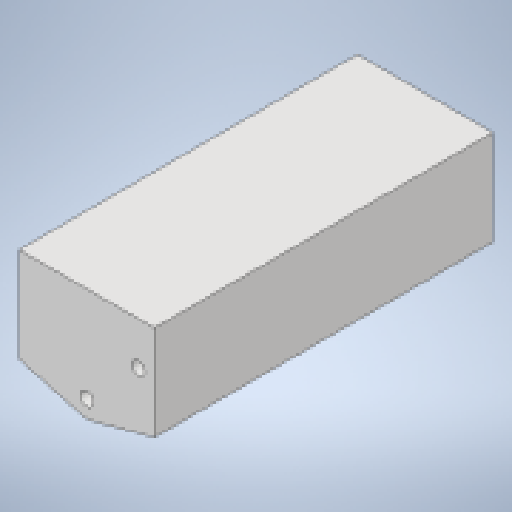
# Autodesk Inventor part: Корпус
Saved by Autodesk Inventor 2025 (Build 290162010, 162A)
## iProperties
Created: 2024-06-14
Part Number: Корпус
Material: Типовые
Document SubType Name: Modeling
Designer: Edward_Higgins
Density: 1 g/cm^3
Appearance: По умолчанию
Author: Edward_Higgins
Autodesk Inventor part; units mm, degrees
ref_plane "YZ Plane" through (0, 0, 0) normal (1, 0, 0) x (0, 1, 0)
ref_plane "XZ Plane" through (0, 0, 0) normal (0, 1, 0) x (-1, 0, 0)
ref_plane "XY Plane" through (0, 0, 0) normal (0, 0, 1) x (1, 0, 0)
sketch "Эскиз1" plane through (0, 0, 0) normal (0, 0, 1) x (1, 0, 0)
  line L0 (-50, 70) -> (50, 70)
  line L1 (50, 70) -> (50, 0)
  line L2 (50, 0) -> (-50, 0) construction
  line L3 (-50, 0) -> (-50, 70)
  circle A0 centre (0, 0) radius 5
  circle A1 centre (38.1838, 38.1838) radius 5
  line L4 (0, 0) -> (38.1838, 38.1838) construction
  line L5 (-50, 0) -> (-3.3494, -12.5)
  arc A2 (-3.3494, -12.5) -> (3.3494, -12.5) centre (0, 0) ccw
  line L6 (3.3494, -12.5) -> (50, 0)
  dimension "d0" = 54
  dimension "d3" = 45
  dimension "d4" = 100
  dimension "d5" = 70
  dimension "d6" = 10
  dimension "d7" = 15
  constraints: 14 end point, 3 centre point, 3 coincident, 2 parallel, 2 point on circle, 2 tangent, 1 equal radius, 1 horizontal, 1 midpoint, 1 perpendicular
  measures "d0" distance of L4.start L4.end
  measures "d3" angle of L2 L4
  measures "d4" distance between parallel lines of L1 L3
  measures "d5" distance from line of point (0, 0) L0
  measures "d6" diameter of A0
  measures "d7" angle of L2 L5
extrude "Выдавливание1" add sketch "Эскиз1" along normal mid plane 130
sketch "Эскиз2" plane through (-50, 0, 65) normal (-1, 0, 0) x (0, 0, 1)
  line L0 (-10.2072, 102.5609) -> (-117.9195, 102.5609)
  line L1 (-117.9195, 102.5609) -> (-117.9195, 10.3029)
  line L2 (-117.9195, 10.3029) -> (-10.2072, 10.3029)
  line L3 (-10.2072, 10.3029) -> (-10.2072, 102.5609)
  point P0 (-65, 0)
  constraints: 8 end point, 2 parallel, 1 horizontal, 1 perpendicular
extrude "Выдавливание2" cut sketch "Эскиз2" against normal blind 166
